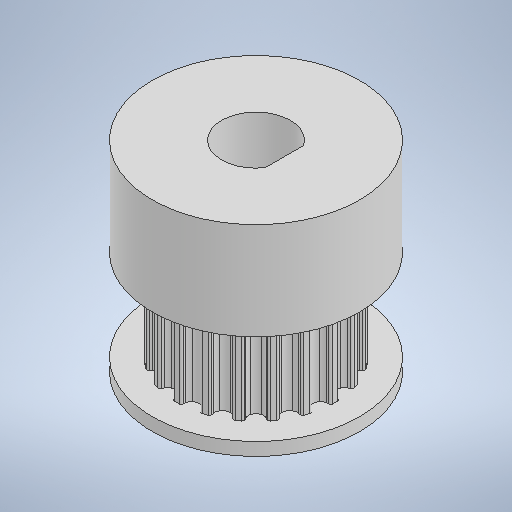
# Autodesk Inventor part: Drive pulley - swivel joint
Saved by Autodesk Inventor 2025.2 (Build 292293000, 293)
## iProperties
Created: 2025-02-03
Part Number: Drive pulley - swivel joint
Material: Generic
Document SubType Name: Modeling
Designer: caomi
Density: 1 g/cm^3
Appearance: Default
Author: caomi
Autodesk Inventor part; units mm, degrees
ref_plane "YZ Plane" through (0, 0, 0) normal (1, 0, 0) x (0, 1, 0)
ref_plane "XZ Plane" through (0, 0, 0) normal (0, 1, 0) x (-1, 0, 0)
ref_plane "XY Plane" through (0, 0, 0) normal (0, 0, 1) x (1, 0, 0)
sketch "Sketch1" plane through (0, 0, 0) normal (0, 1, 0) x (-1, 0, 0)
  circle A0 centre (0, 0) radius 6.3662 construction
  circle A1 centre (0, 0) radius 5.3622 construction
  line L0 (0, 0) -> (6.3662, 0) construction
  line L1 (0, 0) -> (6.2878, -0.9959) construction
  line L2 (0, 0) -> (6.2129, -1.3887) construction
  circle A2 centre (0, 0) radius 6.1122 construction
  line L3 (0, 0) -> (5.3622, 0) construction
  arc A3 (5.4491, -0.5361) -> (5.2962, -0.8388) centre (5.8443, -0.9257) ccw
  arc A4 (5.9601, -0.3333) -> (5.7781, -0.3509) centre (5.965, -1.3333) ccw
  circle A5 centre (0, 0) radius 5.9622 construction
  arc A6 (6.1093, -0.188) -> (6.1122, 0) centre (0, 0) ccw
  line L4 (0, 0) -> (6.1093, -0.188) construction
  line L5 (0, 0) -> (6.1122, 0) construction
  arc A7 (5.9601, -0.3333) -> (6.1093, -0.188) centre (5.9594, -0.1833) ccw
  arc A8 (5.7781, -0.3509) -> (5.4491, -0.5361) centre (5.8888, -0.9327) ccw
  arc A9 (5.2962, 0.8388) -> (5.4491, 0.5361) centre (5.8443, 0.9257) ccw
  arc A10 (5.7781, 0.3509) -> (5.9601, 0.3333) centre (5.965, 1.3333) ccw
  arc A11 (6.1122, 0) -> (6.1093, 0.188) centre (0, 0) ccw
  arc A12 (6.1093, 0.188) -> (5.9601, 0.3333) centre (5.9594, 0.1833) ccw
  arc A13 (5.4491, 0.5361) -> (5.7781, 0.3509) centre (5.8888, 0.9327) ccw
  arc A14 (5.2962, -0.8388) -> (5.2962, 0.8388) centre (0, 0) ccw
  circle A15 centre (0, 0) radius 5.3622
  circle A16 centre (0, 0) radius 6.3662
  circle A17 centre (0, 0) radius 8
  point P0 (5.2962, -0.8388)
  dimension "d0" = 12.7324
  dimension "d1" = 9
  dimension "d2" = 3.6
  dimension "d4" = 1.004
  dimension "d13" = 0.75
  dimension "d14" = 0.555
  dimension "d15" = 1
  dimension "d16" = 0.15
  dimension "d35" = 16
  constraints: 33 point on circle, 17 centre point, 12 end point, 10 coincident, 9 symmetric about line, 6 point on line, 3 tangent, 1 concentric, 1 horizontal, 8 other
  measures "d0" diameter of A0
  measures "d1" angle of L0 L1
  measures "d2" angle of L2 L1
  measures "d4" radial gap between concentric circles of A0 A1
  measures "d13" radial gap between concentric circles of A1 A2
  measures "d14" radius of A3
  measures "d15" radius of A4
  measures "d16" radial gap between concentric circles of A5 A2
  measures "d35" diameter of A17
extrude "Extrusion1" add sketch "Sketch1" along normal blind 4.5 contours A3 A14 A9 A13 A10 A12 A11 A6 A7 A4 A8 | A15 A14 | A16 | A17
extrude "Extrusion2" cut sketch "Sketch1" along normal blind 3.5 contours A3 A14 A9 A13 A10 A12 A11 A6 A7 A4 A8 | A16 | A17
extrude "Extrusion3" add sketch "Sketch1" along normal blind 3.5 contours A3 A14 A9 A13 A10 A12 A11 A6 A7 A4 A8
pattern_circular "Circular Pattern1" count 20 over 360 about axis through (0, 0, 0) along (0, 1, 0) of "Extrusion3"
mirror "Mirror3" about plane through (0, 0, 0) normal (0, -1, 0)
sketch "Sketch2" plane through (0, 4.5, 0) normal (0, 1, 0) x (1, 0, 0)
  circle A0 centre (0, 0) radius 2.65
  line L0 (2.2, 1.4773) -> (2.2, -1.4773)
  dimension "d27" = 5.3
  dimension "d31" = 2.2
  constraints: 2 end point, 2 point on circle, 1 centre point, 1 coincident, 1 vertical
  measures "d27" diameter of A0
  measures "d31" distance from line of point (0, 0) L0
extrude "Extrusion4" cut sketch "Sketch2" against normal through all contours L0 A0 picked at (0.5898, 0.107)
sketch "Sketch3" plane through (0, 3.5, 0) normal (0, -1, 0) x (1, 0, 0)
  circle A0 centre (0, 0) radius 8
  arc A1 (2.2, 1.4773) -> (2.2, -1.4773) centre (0, 0) ccw projected
  line L0 (2.2, -1.4773) -> (2.2, 1.4773) projected
  circle A2 centre (0, 0) radius 8 projected
  constraints: 1 centre point, 1 coincident, 1 concentric
extrude "Extrusion5" add sketch "Sketch3" against normal blind 7.5
equation "\"d0\" = PulleyDia"
equation "\"d1\" = 0.5 * ToothAng"
equation "\"d2\" = TransOffsetAngle"
equation "\"d4\" = PLD + ToothHeight"
equation "\"d13\" = ToothHeight"
equation "\"d14\" = Root_Radius"
equation "\"d15\" = TransRadius"
equation "\"d16\" = Shoulder_Radius"
equation "\"ToothPitch\" = 2"
equation "\"TransOffsetAngle\" = 0.2 * ToothAng"
equation "\"Shoulder_Radius\" = 0.15"
equation "\"Root_Radius\" = 0.555"
equation "\"TransRadius\" = 1"
equation "\"ToothHeight\" = 0.75"
equation "\"PLD\" = 0.254"
equation "\"PulleyDia\" = 12.732395"
equation "\"ToothAng\" = 18deg"
body "Solid1"
